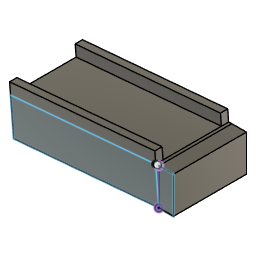
Ramp v2 (Autodesk Fusion 360 design; units mm, degrees)
Autodesk Fusion 360 part; units mm, degrees
sketch "Sketch1" plane through (0, 0, 0) normal (0, 1, 0) x (1, 0, 0)
  line L0 (0, 0) -> (-50.6067, 4.4275)
  line L1 (-50.6067, 4.4275) -> (-51.7136, -8.2242)
  line L2 (-51.7136, -8.2242) -> (-1.1069, -12.6517)
  line L3 (-1.1069, -12.6517) -> (0, 0)
  line L4 (0, 0) -> (5.08, 0)
  line L5 (5.08, 0) -> (5.08, -12.7)
  line L6 (0, -12.7) -> (0, 0)
  line L7 (5.08, -12.7) -> (-0.5534, -12.7) construction
  line L8 (5.08, -12.7) -> (0, -12.7)
  dimension "d4" = 50.8
  dimension "d5" = 12.7
  constraint coincident L0.start L3.end
  constraint horizontal L4
  constraint vertical L5
  constraint vertical L6
  constraint perpendicular L6 L7
  constraint coincident L7 L6.start
  measures "d4" distance of L0.start L0.end
  measures "d5" distance of L0.end L1.end
extrude "Extrude1" add sketch "Sketch1" along normal blind 25.4 contours L0 L1 L2 L3 makes body 1
sketch "Sketch2" plane through (0, 0, 0) normal (0, 1, 0) x (1, 0, 0)
  line L0 (0, -12.7) -> (0, 0)
  line L1 (-1.1069, -12.6517) -> (0, -12.7485)
  point P0 (-1.1069, -12.6517)
  constraint coincident P0 L1.start
  constraint coincident L0 L1.end
extrude "Extrude3" add sketch "Sketch1" along normal blind 25.4 separate body contours L4 L5 L6 L8 makes body 2
loft "Loft1" add section 1 face at (0, 8.4667, 8.4667) section 2 face at (-0.7379, 8.4667, 8.4344) separate body on bodies 1 2 makes body 3
sketch "Sketch3" plane through (0, 0, 0) normal (0, 0, 1) x (1, 0, 0)
sketch "Sketch4" plane through (-1.1069, 0, 12.6517) normal (-0.087156, 0, 0.996195) x (0, -1, 0)
  line L0 (0, -50.8) -> (0, 0)
  line L1 (0, 0) -> (-25.4, 0)
  line L2 (-25.4, 0) -> (-25.4, -50.8)
  line L3 (-25.4, -50.8) -> (0, -50.8)
  line L4 (0, 0) -> (-2.54, 0)
  line L5 (-2.54, 0) -> (-2.54, -50.8)
  line L6 (-2.54, -50.8) -> (0, -50.8)
  line L7 (0, -50.8) -> (0, 0)
  line L8 (-2.54, -48.26) -> (-25.4, -48.26)
  line L9 (-25.4, -48.26) -> (-25.4, -50.8)
  line L10 (-25.4, -50.8) -> (-2.54, -50.8)
  line L11 (-2.54, -50.8) -> (-2.54, -48.26)
  line L12 (-25.4, -50.8) -> (-22.86, -50.8)
  line L13 (-22.86, -50.8) -> (-22.86, 0)
  line L14 (-22.86, 0) -> (-25.4, 0)
  line L15 (-25.4, 0) -> (-25.4, -50.8)
  dimension "d18" = 50.8
  dimension "d19" = 2.54
  dimension "d20" = 50.8
  dimension "d21" = 2.54
  dimension "d22" = 2.54
  constraint horizontal L4
  constraint vertical L5
  constraint horizontal L6
  constraint vertical L7
  constraint coincident L3 L5.end
  constraint coincident L0.end L1.start
  constraint horizontal L8
  constraint vertical L9
  constraint horizontal L10
  constraint vertical L11
  constraint coincident L2.end L3.start
  constraint horizontal L12
  constraint vertical L13
  constraint horizontal L14
  constraint vertical L15
  constraint coincident L1 L13.end
  measures "d18" distance of L4.end L5.end
  measures "d19" distance of L5.end L0.start
  measures "d20" distance of L12.end L13.end
  measures "d21" distance of L13.end L1.end
  measures "d22" distance of L8 L10
extrude "Extrude4" add sketch "Sketch4" along normal blind 3.81 contours L0 L1 L3 L4 L5 L6 L7 L11 | L2 L3 L8 L9 L10 L12 L13 L15 | L1 L2 L8 L13 L14 L15 bodies 1 3
equation "length = 2 in"
equation "height = 0.5 in"
equation "depression = -5 deg"
equation "d4 = length"
equation "d5 = height"
equation "width = 1 in"
equation "d10 = width"
equation "d15 = width"
equation "wallWidth = 0.1 in"
equation "d19 = wallWidth"
equation "d21 = wallWidth"
equation "d22 = wallWidth"
equation "wallHeight = 0.15 in"
equation "d24 = wallHeight"
